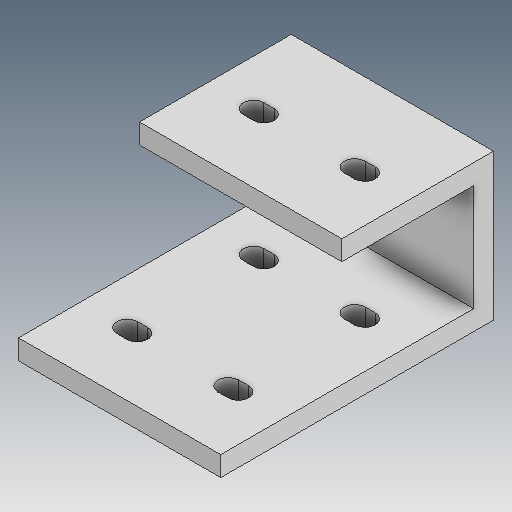
# Autodesk Inventor part: hanging_bracket_t-slot-2inx1in
Saved by Autodesk Inventor 2025.1 (Build 291241000, 241)
## iProperties
Created: 2026-07-04
Part Number: hanging_bracket_t-slot-2inx1in
Material: Generic
Document SubType Name: Modeling
Designer: Aiden
Density: 1 g/cm^3
Appearance: Default
Author: Aiden
Autodesk Inventor part; units mm, degrees
ref_plane "YZ Plane" through (0, 0, 0) normal (1, 0, 0) x (0, 1, 0)
ref_plane "XZ Plane" through (0, 0, 0) normal (0, 1, 0) x (-1, 0, 0)
ref_plane "XY Plane" through (0, 0, 0) normal (0, 0, 1) x (1, 0, 0)
sketch "Sketch1" plane through (0, 0, 0) normal (0, 1, 0) x (-1, 0, 0)
  line L0 (25.4, 31.75) -> (-25.4, 31.75)
  line L1 (-25.4, 31.75) -> (-25.4, -31.75)
  line L2 (-25.4, -31.75) -> (25.4, -31.75)
  line L3 (25.4, -31.75) -> (25.4, 31.75)
  line L4 (25.4, 31.75) -> (-25.4, -31.75) construction
  line L5 (-25.4, 31.75) -> (25.4, -31.75) construction
  point P0 (0, 0)
  dimension "d0" = 50.8
  dimension "d1" = 63.5
  constraints: 12 end point, 2 midpoint, 2 parallel, 1 horizontal, 1 perpendicular
  measures "d0" distance of L0.start L0.end
  measures "d1" distance of L0.end L1.end
extrude "Extrusion1" add sketch "Sketch1" along normal blind 5
sketch "Sketch2" plane through (0, 5, 0) normal (0, 1, 0) x (1, 0, 0)
  line L0 (25.4, 31.75) -> (-25.4, 31.75) construction
  line L1 (-25.4, -31.75) -> (25.4, -31.75) construction
  line L2 (-25.4, 31.75) -> (-25.4, -31.75) construction
  line L3 (-25.4, 0) -> (25.4, 0) construction
  line L4 (25.4, -31.75) -> (25.4, 31.75) construction
  line L5 (0, 31.75) -> (0, 0) construction
  line L6 (0, 0) -> (0, -31.75) construction
  line L7 (0, 15.875) -> (-25.4, 15.875) construction
  line L8 (-13.97, 15.875) -> (-11.43, 15.875) construction
  line L9 (-13.97, 13.275) -> (-11.43, 13.275)
  line L10 (-11.43, 18.475) -> (-13.97, 18.475)
  arc A0 (-13.97, 18.475) -> (-13.97, 13.275) centre (-13.97, 15.875) ccw
  arc A1 (-11.43, 13.275) -> (-11.43, 18.475) centre (-11.43, 15.875) ccw
  line L11 (0, 15.875) -> (25.4, 15.875) construction
  line L12 (13.97, 13.275) -> (11.43, 13.275)
  line L13 (11.43, 18.475) -> (13.97, 18.475)
  arc A2 (13.97, 13.275) -> (13.97, 18.475) centre (13.97, 15.875) ccw
  arc A3 (11.43, 18.475) -> (11.43, 13.275) centre (11.43, 15.875) ccw
  line L14 (-13.97, -13.275) -> (-11.43, -13.275)
  line L15 (-11.43, -18.475) -> (-13.97, -18.475)
  arc A4 (-13.97, -13.275) -> (-13.97, -18.475) centre (-13.97, -15.875) ccw
  arc A5 (-11.43, -18.475) -> (-11.43, -13.275) centre (-11.43, -15.875) ccw
  arc A6 (11.43, -13.275) -> (11.43, -18.475) centre (11.43, -15.875) ccw
  line L16 (13.97, -13.275) -> (11.43, -13.275)
  line L17 (11.43, -18.475) -> (13.97, -18.475)
  arc A7 (13.97, -18.475) -> (13.97, -13.275) centre (13.97, -15.875) ccw
  point P0 (-12.7, 15.875)
  point P1 (-12.7, 13.275)
  point P2 (-12.7, 18.475)
  dimension "d4" = 11.43
  dimension "d5" = 13.97
  dimension "d6" = 5.2
  constraints: 30 end point, 19 symmetric about line, 16 point on circle, 8 centre point, 8 midpoint, 5 point on line, 4 tangent, 2 perpendicular, 1 collinear, 1 parallel, 6 other
  measures "d4" distance from line of L5 L8.end
  measures "d5" distance from line of L5 L8.start
  measures "d6" distance of point (-12.7, 13.275) point (-12.7, 18.475)
extrude "Extrusion2" cut sketch "Sketch2" against normal blind 5
sketch "Sketch3" plane through (25.4, 0, -31.75) normal (0, 0, -1) x (-1, 0, 0)
  line L0 (0, 0) -> (50.8, 0) construction
  line L1 (50.8, 0) -> (0, 0)
  line L2 (0, 0) -> (0, 31.75)
  line L3 (0, 31.75) -> (50.8, 31.75)
  line L4 (50.8, 31.75) -> (50.8, 0)
  point P0 (25.4, 0)
  dimension "d9" = 31.75
  constraints: 8 end point, 2 parallel, 1 horizontal, 1 perpendicular, 1 point on line
  measures "d9" distance of L3.end L0.end
extrude "Extrusion3" add sketch "Sketch3" along normal blind 5
sketch "Sketch4" plane through (-25.4, 31.75, -31.75) normal (0, 1, 0) x (1, 0, 0)
  line L0 (0, 5) -> (50.8, 5) construction
  line L1 (50.8, -63.5) -> (50.8, 0) construction
  line L2 (0, 5) -> (50.8, 5)
  line L3 (50.8, 5) -> (50.8, -33.1)
  line L4 (50.8, -33.1) -> (0, -33.1)
  line L5 (0, -33.1) -> (0, 5)
  point P0 (25.4, -31.75)
  dimension "d12" = 38.1
  constraints: 8 end point, 2 parallel, 1 horizontal, 1 perpendicular, 1 point on line
  measures "d12" distance of L4.end L0.start
extrude "Extrusion4" add sketch "Sketch4" along normal blind 5
sketch "Sketch5" plane through (-25.4, 36.75, -31.75) normal (0, 1, 0) x (1, 0, 0)
  line L0 (39.37, -50.225) -> (36.83, -50.225) construction
  arc A0 (36.83, -45.025) -> (36.83, -50.225) centre (36.83, -47.625) ccw construction
  line L1 (36.83, -45.025) -> (39.37, -45.025) construction
  arc A1 (39.37, -50.225) -> (39.37, -45.025) centre (39.37, -47.625) ccw construction
  arc A2 (36.83, -13.275) -> (36.83, -18.475) centre (36.83, -15.875) ccw projected
  line L2 (36.83, -13.275) -> (39.37, -13.275) projected
  arc A3 (39.37, -18.475) -> (39.37, -13.275) centre (39.37, -15.875) ccw projected
  line L3 (39.37, -18.475) -> (36.83, -18.475) projected
  arc A4 (11.43, -45.025) -> (11.43, -50.225) centre (11.43, -47.625) ccw construction
  line L4 (11.43, -45.025) -> (13.97, -45.025) construction
  arc A5 (13.97, -50.225) -> (13.97, -45.025) centre (13.97, -47.625) ccw construction
  line L5 (13.97, -50.225) -> (11.43, -50.225) construction
  line L6 (11.43, -13.275) -> (13.97, -13.275) projected
  arc A6 (13.97, -18.475) -> (13.97, -13.275) centre (13.97, -15.875) ccw projected
  line L7 (13.97, -18.475) -> (11.43, -18.475) projected
  arc A7 (11.43, -13.275) -> (11.43, -18.475) centre (11.43, -15.875) ccw projected
  line L8 (50.8, -63.5) -> (50.8, 0) construction
  line L9 (50.8, 0) -> (0, 0) construction
  line L10 (0, 0) -> (0, -63.5) construction
  line L11 (0, -63.5) -> (50.8, -63.5) construction
  point P0 (25.4, -31.75)
extrude "Extrusion5" cut sketch "Sketch5" against normal blind 5
body "Solid1"
